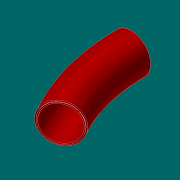
# Autodesk Inventor part: A1-19027-100-04 HCWI elbow - male
Saved by Autodesk Inventor 2017.3 (Build 213257000, 257)
## iProperties
Created: 2019-06-26
Part Number: A1-19027-100-04 HCWI elbow - male
Material: Iron, HCWI
Document SubType Name: Modeling
Designer: Graeme_Van_Dongen
Density: 7.33517 g/cm^3
Appearance: Iron Gray(1)
Mass: 1.94047e+06 g
Surface Area: 107204 cm^2
Volume: 264543 cm^3
Description: 28 1/2" ID x 2" WALL x 30° HCWI ELBOW - MALE, ASTM A532 CLASS III TYPE A, PF# 470284
Author: Graeme_Van_Dongen
Autodesk Inventor part; units mm, degrees
ref_plane "YZ Plane" through (0, 0, 0) normal (1, 0, 0) x (0, 1, 0)
ref_plane "XZ Plane" through (0, 0, 0) normal (0, 1, 0) x (-1, 0, 0)
ref_plane "XY Plane" through (0, 0, 0) normal (0, 0, 1) x (1, 0, 0)
sketch "Sketch1" plane through (0, 0, 0) normal (0, 0, 1) x (1, 0, 0)
  circle A0 centre (-4064, 0) radius 361.95
  circle A1 centre (-4064, 0) radius 412.75
  line L0 (0, -577.85) -> (0, 577.85) projected
  point P0 (0, 0)
  dimension "d0" = 723.9
  dimension "d1" = 825.5
  dimension "d2" = 4064
  constraints: 2 centre point, 1 coincident, 1 horizontal alignment
  measures "d0" diameter of A0
  measures "d1" diameter of A1
  measures "d2" distance of point (0, 0) A0.centre
revolve "Revolution1" add sketch "Sketch1" angle 30 about axis through (0, -10, 0) along (0, 1, 0)
sketch "Sketch10" plane through (-4064, 0, 0) normal (0, 0, -1) x (-1, 0, 0)
  circle A0 centre (0, 0) radius 387.35
  circle A1 centre (0, 0) radius 412.75 construction
  point P0 (-4064, 0)
  dimension "d34" = 774.7
  constraints: 1 centre point, 1 coincident
  measures "d34" diameter of A0
extrude "Extrusion9" cut sketch "Sketch10" against normal blind 12.7
sketch "Sketch11" plane through (-3519.5272, 0, 2032) normal (0.5, 0, 0.8660254) x (0.8660254, 0, -0.5)
  circle A0 centre (0, 0) radius 361.95 projected
  circle A1 centre (0, 0) radius 387.096
  circle A2 centre (0, 0) radius 425.45
  line L0 (4064, -595.63) -> (4064, 595.63) projected
  point P0 (4064, 0)
  dimension "d37" = 774.192
  dimension "d38" = 850.9
  constraints: 2 centre point, 2 coincident
  measures "d37" diameter of A1
  measures "d38" diameter of A2
extrude "Extrusion10" cut sketch "Sketch11" against normal blind 6.35 contours A2
extrude "Extrusion11" add sketch "Sketch11" along normal blind 6.35 contours A0 | A1
revolve "Revolution2" cut sketch "Sketch11" angle 0.5 about axis through (0, -10, 0) along (0, 1, 0) contours A0
fillet "Fillet3" radius 0.7937 2 edges at (-3857.9382, 0, 2220.047) (-3676.65, 0, 12.7)
chamfer "Chamfer3" distance 0.7937 angle 45 2 edges at (-3851.5872, 0, 2231.0473) (-3676.65, 0, 0)
body "Solid1"
